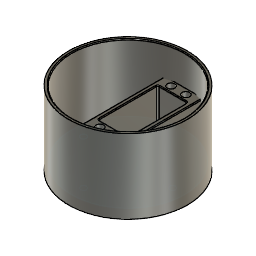
rotating base bottom v2 (Autodesk Fusion 360 design; units mm, degrees)
Autodesk Fusion 360 part; units mm, degrees
note: some values were not read from the file. Set by a fixed rule: which sketch regions a step uses.
sketch "Sketch1" plane through (0, 0, 0) normal (0, 0, 1) x (1, 0, 0)
  circle A0 centre (0, 0) radius 40
  constraint coincident A0.centre origin
extrude "Extrude1" add sketch "Sketch1" along normal blind 5 makes body 1
sketch "Sketch2" plane through (0, 0, 5) normal (0, 0, 1) x (-1, 0, 0)
  circle A0 centre (0, 0) radius 40
  circle A1 centre (0, 0) radius 38
  dimension "d3" = 76
  constraint concentric A0 A1
  measures "d3" diameter of A1
extrude "Extrude2" add sketch "Sketch2" along normal blind 45 bodies 1
sketch "Sketch3" plane through (0, 0, 5) normal (0, 0, 1) x (-1, 0, 0)
  circle A0 centre (0, 0) radius 38
  circle A1 centre (0, -30) radius 2
  circle A2 centre (0, 0) radius 30
  circle A3 centre (-30, 0) radius 2
  circle A4 centre (0, 30) radius 2
  circle A5 centre (30, 0) radius 2
  circle A6 centre (0, 0) radius 10
  circle A7 centre (0, -10) radius 2
  circle A8 centre (-10, 0) radius 2
  circle A9 centre (0, 10) radius 2
  circle A10 centre (10, 0) radius 2
  circle A11 centre (0, 0) radius 20
  circle A12 centre (0, -20) radius 2
  circle A13 centre (-20, 0) radius 2
  circle A14 centre (0, 20) radius 2
  circle A15 centre (20, 0) radius 2
  point P0 (0, -6.5)
  constraint concentric A0 A2
  constraint coincident A1.centre A2
  constraint coincident A2 A3.centre
  constraint coincident A2 A4.centre
  constraint coincident A2 A5.centre
  constraint concentric A2 A6
  constraint coincident A6 A7.centre
  constraint coincident A6 A8.centre
  constraint coincident A6 A9.centre
  constraint coincident A6 A10.centre
  constraint concentric A2 A11
  constraint coincident A11 A12.centre
  constraint coincident A11 A13.centre
  constraint coincident A11 A14.centre
  constraint coincident A11 A15.centre
sketch "Sketch4" plane through (0, 0, 5) normal (0, 0, 1) x (-1, 0, 0)
  line L0 (0, 0) -> (0, -30)
  line L1 (0, 0) -> (0, 10)
  line L2 (0, 10) -> (-10, 10)
  line L3 (-10, 10) -> (10, 10)
  line L4 (10, 10) -> (11, 10)
  line L5 (11, 10) -> (-11, 10)
  line L6 (10, 10) -> (-10, 10)
  line L7 (-10, 10) -> (-10, -30)
  line L8 (-10, -30) -> (10, -30)
  line L9 (10, -30) -> (10, 10)
  line L10 (0, -30) -> (0, -37.5)
  line L11 (0, 10) -> (-3, 10)
  line L12 (-3, 10) -> (-3, 17.5)
  line L13 (-3, 17.5) -> (0, 17.5)
  line L14 (0, 17.5) -> (0, 10)
  line L15 (12.8457, -37.5) -> (-13, -37.5)
  line L16 (-13, -37.5) -> (-13, 18)
  line L17 (-13, 18) -> (12.8457, 18)
  line L18 (12.8457, 18) -> (12.8457, -37.5)
  dimension "d6" = 30
  dimension "d7" = 10
  dimension "d8" = 7.5
  dimension "d9" = 7.5
  constraint coincident L0.start L1.start
  constraint vertical L0
  constraint parallel L0 L1
  constraint perpendicular L1 L2
  constraint perpendicular L1 L3
  constraint perpendicular L1 L4
  constraint parallel L3 L5
  constraint horizontal L6
  constraint vertical L7
  constraint horizontal L8
  constraint vertical L9
  constraint perpendicular L8 L10
  constraint horizontal L11
  constraint vertical L12
  constraint horizontal L13
  constraint vertical L14
  constraint horizontal L15
  constraint vertical L16
  constraint horizontal L17
  constraint vertical L18
  measures "d6" distance of L0.start L0.end
  measures "d7" distance of L1.end L0.start
  measures "d8" distance of L0.end L10.end
  measures "d9" distance of L1.end L13.end
extrude "Extrude3" add sketch "Sketch4" along normal blind 25 separate body contours L2 L3 L5 L6 L11 L12 L13 L14 | L15 L16 L17 L18 makes body 2
fillet "Fillet1" radius 1 4 edges at (-10, 30, 17.5) (10, 30, 17.5) (-10, -10, 17.5) (10, -10, 17.5) on bodies 2
sketch "Sketch5" plane through (0, 0, 30) normal (0, 0, 1) x (-1, 0, 0)
  line L0 (-9, 10) -> (9, 10)
  arc A0 (10, 9) -> (9, 10) centre (9, 9) ccw
  line L1 (10, 9) -> (10, -29)
  arc A1 (9, -30) -> (10, -29) centre (9, -29) ccw
  line L2 (9, -30) -> (-9, -30)
  arc A2 (-10, -29) -> (-9, -30) centre (-9, -29) ccw
  line L3 (-10, -29) -> (-10, 9)
  arc A3 (-9, 10) -> (-10, 9) centre (-9, 9) ccw
  line L4 (12.8457, 18) -> (-13, 18)
  line L5 (-13, 18) -> (-13, -37.5)
  line L6 (-13, -37.5) -> (12.8457, -37.5)
  line L7 (12.8457, -37.5) -> (12.8457, 18)
  line L8 (0, 0) -> (-5, 0)
  line L9 (-5, 0) -> (0, 0)
  line L10 (4, 0) -> (0, 0)
  line L11 (5, 0) -> (4, 0)
  line L12 (-5, 14) -> (5, 14)
  line L13 (5, 14) -> (5, -34)
  line L14 (5, -34) -> (-5, -34)
  line L15 (-5, -34) -> (-5, 14)
  circle A4 centre (5, -34) radius 2.5
  circle A5 centre (-5, -34) radius 2.5
  circle A6 centre (5, 14) radius 2.5
  circle A7 centre (-5, 14) radius 2.5
  dimension "d14" = 5
  dimension "d15" = 5
  dimension "d16" = 5
  dimension "d17" = 5
  constraint coincident L8.start L9.end
  constraint horizontal L8
  constraint parallel L8 L10
  constraint parallel L10 L11
  constraint horizontal L12
  constraint vertical L13
  constraint horizontal L14
  constraint vertical L15
  constraint coincident L13.end L14.start
  constraint coincident L14.end L15.start
  constraint coincident L12.end L13.start
  constraint coincident L12.start L15.end
  measures "d14" diameter of A4
  measures "d15" diameter of A5
  measures "d16" diameter of A6
  measures "d17" diameter of A7
extrude "Extrude4" cut sketch "Sketch5" against normal blind 20 contours L12 L15 A7 | L12 L15 A7 | L12 L13 A6 | L12 L13 A6 | L14 L15 A5 | L14 L15 A5 | L13 L14 A4 | L13 L14 A4 bodies 2
extrude "Extrude5" cut sketch "Sketch3" against normal blind 10 contours A2 A5 | A2 A5 | A2 A3 | A2 A3 | A2 A4 | A2 A4 bodies 1
fillet "Fillet2" radius 0.5 11 edges at (0.0772, -18, 30) (-12.8457, 9.75, 30) (13, 9.75, 30) (9.7071, -9.7071, 30) (0, -10, 30) (-9.7071, -9.7071, 30) (-10, 10, 30) (-9.7071, 29.7071, 30) (0, 30, 30) (9.7071, 29.7071, 30) (10, 10, 30) on bodies 2
fillet "Fillet3" radius 0.5 1 edges at (35.4284, -13.7414, 50) on bodies 1
sketch "Sketch6" plane through (0, 0, 5) normal (0, 0, 1) x (-1, 0, 0)
  circle A0 centre (30, 0) radius 2
  circle A1 centre (0, 30) radius 2
  circle A2 centre (-30, 0) radius 2
  circle A3 centre (0, 0) radius 38
  circle A4 centre (0, 0) radius 40
  circle A5 centre (0, 0) radius 40
  circle A6 centre (0, 0) radius 40
  dimension "d26" = 80
  dimension "d27" = 80
  dimension "d28" = 80
  constraint coincident A3.centre A4.centre
  measures "d26" diameter of A5
  measures "d27" diameter of A6
  measures "d28" diameter of A5
sketch "Sketch7" plane through (0, 0, 5) normal (0, 0, 1) x (-1, 0, 0)
sketch "Sketch8" plane through (0, 0, 0) normal (0, 1, 0) x (1, 0, 0)
  line L0 (38, -49.5) -> (-38, -49.5)
  line L1 (0, -5) -> (-6, -5)
  line L2 (-6, -5) -> (-6, -9)
  line L3 (-6, -9) -> (0, -9)
  line L4 (0, -9) -> (0, -5)
  line L5 (0, -5) -> (6, -5)
  line L6 (6, -5) -> (6, -9)
  line L7 (6, -9) -> (0, -9)
  line L8 (0, -9) -> (0, -5)
  line L9 (6, -9) -> (-6, -9)
  line L10 (-6, -9) -> (-6, -27)
  line L11 (-6, -27) -> (6, -27)
  line L12 (6, -27) -> (6, -9)
  dimension "d29" = 49.5
  constraint horizontal L1
  constraint vertical L2
  constraint horizontal L3
  constraint vertical L4
  constraint horizontal L5
  constraint vertical L6
  constraint horizontal L7
  constraint vertical L8
  constraint horizontal L9
  constraint vertical L10
  constraint horizontal L11
  constraint vertical L12
  measures "d29" distance of origin L0
extrude "Extrude6" cut sketch "Sketch8" against normal blind 43 contours L1 L2 L3 L4 L8 L9 | L4 L5 L6 L7 L8 L9 bodies 2
sketch "Sketch9" plane through (0, 0, 0) normal (0, 1, 0) x (1, 0, 0)
  line L0 (0, -5) -> (6, -5)
  line L1 (6, -5) -> (6, -9)
  line L2 (6, -9) -> (0, -9)
  line L3 (0, -9) -> (0, -5)
  line L4 (0, -5) -> (-6, -5)
  line L5 (-6, -5) -> (-6, -9)
  line L6 (-6, -9) -> (0, -9)
  line L7 (0, -9) -> (0, -5)
  line L8 (6, -9) -> (-6, -9)
  line L9 (-6, -9) -> (-6, -27)
  line L10 (-6, -27) -> (6, -27)
  line L11 (6, -27) -> (6, -9)
  constraint horizontal L0
  constraint vertical L1
  constraint horizontal L2
  constraint vertical L3
  constraint horizontal L4
  constraint vertical L5
  constraint horizontal L6
  constraint vertical L7
  constraint horizontal L8
  constraint vertical L9
  constraint horizontal L10
  constraint vertical L11
extrude "Extrude7" cut sketch "Sketch9" against normal blind 20 contours L2 L6 L8 L9 L10 L11 bodies 2
sketch "Sketch10" plane through (0, 0, 5) normal (0, 0, 1) x (-1, 0, 0)
  circle A0 centre (30, 0) radius 2
  circle A1 centre (0, 30) radius 2
  circle A2 centre (-30, 0) radius 2
  circle A3 centre (0, 0) radius 38
sketch "Sketch11" plane through (0, 0, 5) normal (0, 0, 1) x (-1, 0, 0)
  circle A0 centre (0, 0) radius 30
  line L0 (0, 0) -> (-6, 0)
  line L1 (-6, 0) -> (0, 0)
  line L2 (0, 5) -> (0, 0)
  line L3 (0, 0) -> (-70.7107, 70.7107)
  circle A1 centre (-21.2132, 21.2132) radius 7.5
  dimension "d34" = 100
  dimension "d35" = 45
  dimension "d36" = 15
  constraint coincident A0.centre L0.start
  constraint horizontal L0
  constraint perpendicular L1 L2
  constraint coincident L3 A1.centre
  constraint coincident A0 A1.centre
  measures "d34" distance of A0.centre L3.end
  measures "d35" angle of L2 L3
  measures "d36" diameter of A1
extrude "Extrude8" cut sketch "Sketch11" against normal blind 100 contours A0 L3 A1 | A0 L3 A1 | A0 L3 A1 | A0 L3 A1 bodies 1
